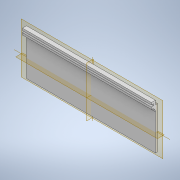
# Autodesk Inventor part: Hanging_Wall
Saved by Autodesk Inventor 2022.4 (Build 264492010, 492A)
## iProperties
Created: 2025-02-20
Part Number: Hanging_Wall
Material: Generic
Document SubType Name: Modeling
Designer: jan-m
Density: 1 g/cm^3
Appearance: Default
Author: jan-m
Autodesk Inventor part; units mm, degrees
sketch "Sketch2" plane through (0, 0, 0) normal (1, 0, 0) x (0, 1, 0)
  line L0 (13.85, 0.8) -> (-13.85, 0.8)
  line L1 (-13.85, 0.8) -> (-13.85, -0.8)
  line L2 (-13.85, -0.8) -> (18.65, -0.8)
  line L3 (18.65, -0.8) -> (18.65, 0.8)
  line L4 (0, 4.96) -> (0, -1.76) projected
  line L5 (-20.95, 0) -> (28.75, 0) projected
  line L6 (18.65, 0.8) -> (21.65, 0.8)
  line L7 (21.65, 0.8) -> (21.65, 4)
  line L8 (21.65, 4) -> (20.05, 4)
  line L9 (20.05, 4) -> (20.05, 2.4)
  line L10 (20.05, 2.4) -> (18.65, 2.4)
  line L11 (18.65, 2.4) -> (18.65, 4)
  line L12 (18.65, 4) -> (17.05, 4)
  line L13 (17.05, 4) -> (17.05, 4)
  arc A0 (13.85, 0.8) -> (17.05, 4) centre (13.85, 4) ccw
  point P0 (0, 0)
  point P1 (0, 0.8)
  point P2 (18.65, 0)
  dimension "d0" = 32.5
  dimension "d1" = 1.6
  dimension "d2" = 3
  dimension "d3" = 3.2
  dimension "d4" = 1.6
  dimension "d6" = 1.6
  dimension "d7" = 1.6
  dimension "d8" = 1.4
  dimension "d12" = 1.6
  dimension "d13" = 3.2
  constraints: 24 end point, 7 perpendicular, 3 horizontal, 3 point on line, 2 midpoint, 2 parallel, 2 point on circle, 1 centre point
  measures "d0" distance of L2.end L1.end
  measures "d1" distance of L2.end L3.end
  measures "d2" distance of L3.end L6.end
  measures "d3" distance of L6.end L7.end
  measures "d4" distance of L7.end L8.end
  measures "d6" distance of L11.end L12.end
  measures "d7" distance of L10.end L11.end
  measures "d8" distance between parallel lines of L9 L11
  measures "d12" distance between parallel lines of L6 L10
  measures "d13" radius of A0
extrude "Extrusion1" add sketch "Sketch2" along normal mid plane 100
equation "\"d13\" = d3"
body "Solid1"
